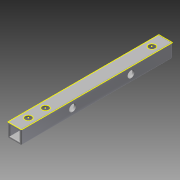
# Autodesk Inventor part: Vertical Rod
Saved by Autodesk Inventor 2013 (Build 170138000, 138)
## iProperties
Created: 2014-05-22
Part Number: Vertical Rod
Material: Steel
Document SubType Name: Modeling
Designer: ryclifton
Mass: 683.775 g
Surface Area: 479.026 cm^2
Volume: 87.105 cm^3
Density: 7.85 g/cm^3
Author: ryclifton
Autodesk Inventor part; units mm, degrees
ref_plane "YZ Plane" through (0, 0, 0) normal (1, 0, 0) x (0, 1, 0)
ref_plane "XZ Plane" through (0, 0, 0) normal (0, 1, 0) x (-1, 0, 0)
ref_plane "XY Plane" through (0, 0, 0) normal (0, 0, 1) x (1, 0, 0)
sketch "Sketch1" plane through (0, 0, 0) normal (0, 0, 1) x (1, 0, 0)
  line L0 (0, 0) -> (25.4, 0)
  line L1 (25.4, 0) -> (25.4, 25.4)
  line L2 (25.4, 25.4) -> (0, 25.4)
  line L3 (0, 25.4) -> (0, 0)
  dimension "d0" = 25.4
  dimension "d1" = 25.4
  constraints: 8 end point, 2 parallel, 1 horizontal, 1 perpendicular
  measures "d0" distance of L2.end L1.end
  measures "d1" distance of L1.end L0.end
extrude "Extrusion1" add sketch "Sketch1" along normal blind 279.4
sketch "Sketch2" plane through (0, 25.4, 0) normal (0, 1, 0) x (1, 0, 0)
  line L0 (0, 0) -> (0, -279.4) projected
  line L1 (25.4, 0) -> (25.4, -279.4) projected
  line L2 (0, 0) -> (0, -25.4)
  line L3 (0, -25.4) -> (12.7, -25.4)
  circle A0 centre (12.7, -25.4) radius 6.35
  line L4 (25.4, -279.4) -> (25.4, -254)
  line L5 (25.4, -254) -> (12.7, -254)
  circle A1 centre (12.7, -254) radius 6.35
  dimension "d4" = 25.4
  dimension "d5" = 12.7
  dimension "d6" = 25.4
  dimension "d7" = 12.7
  constraints: 8 end point, 2 centre point, 2 coincident, 2 perpendicular, 2 point on line
  measures "d4" distance of L0.start L2.end
  measures "d5" diameter of A0
  measures "d6" distance of L1.end L4.end
  measures "d7" diameter of A1
extrude "Extrusion2" cut sketch "Sketch2" against normal blind 279.4
sketch "Sketch3" plane through (0, 0, 0) normal (0, 0, -1) x (-1, 0, 0)
  line L0 (0, 0) -> (-25.4, 0) projected
  line L1 (-25.4, 25.4) -> (0, 25.4) projected
  line L2 (-25.4, 0) -> (-25.4, 25.4) projected
  line L3 (-25.4, 25.4) -> (-25.4, 21.59)
  line L4 (-25.4, 21.59) -> (-21.59, 21.59)
  line L5 (-25.4, 0) -> (-21.59, 0)
  line L6 (-21.59, 0) -> (-21.59, 3.81)
  line L7 (0, 0) -> (-3.81, 0)
  line L8 (-3.81, 0) -> (-3.81, 3.81)
  line L9 (0, 25.4) -> (-3.81, 25.4)
  line L10 (-3.81, 25.4) -> (-3.81, 21.59)
  line L11 (-3.81, 21.59) -> (-21.59, 21.59)
  line L12 (-21.59, 21.59) -> (-21.59, 3.81)
  line L13 (-21.59, 3.81) -> (-3.81, 3.81)
  line L14 (-3.81, 3.81) -> (-3.81, 21.59)
  dimension "d10" = 3.81
  dimension "d11" = 3.81
  dimension "d12" = 3.81
  dimension "d13" = 3.81
  dimension "d14" = 3.81
  dimension "d15" = 3.81
  dimension "d16" = 3.81
  dimension "d17" = 3.81
  constraints: 24 end point, 4 perpendicular, 4 point on line
  measures "d10" distance of L1.start L3.end
  measures "d11" distance of L3.end L4.end
  measures "d12" distance of L0.end L5.end
  measures "d13" distance of L5.end L6.end
  measures "d14" distance of L0.start L7.end
  measures "d15" distance of L7.end L8.end
  measures "d16" distance of L1.end L9.end
  measures "d17" distance of L9.end L10.end
extrude "Extrusion3" cut sketch "Sketch3" against normal blind 279.4 contours L13 L12 L11 L14
sketch "Sketch4" plane through (0, 0, 0) normal (0, -1, 0) x (1, 0, 0)
  circle A0 centre (12.7, 254) radius 6.35 projected
  line L0 (0, 0) -> (0, 279.4) projected
  line L1 (12.7, 247.65) -> (12.7, 222.25)
  circle A1 centre (12.7, 222.25) radius 6.35
  dimension "d20" = 25.4
  dimension "d21" = 12.7
  constraints: 2 end point, 1 centre point, 1 coincident, 1 parallel, 1 vertical alignment, 1 other
  measures "d20" distance of L1.start L1.end
  measures "d21" diameter of A1
extrude "Extrusion4" cut sketch "Sketch4" against normal blind 279.4 contours A1
sketch "Sketch5" plane through (0, 25.4, 0) normal (0, 1, 0) x (1, 0, 0)
  circle A0 centre (12.7, -222.25) radius 6.35 projected
  circle A1 centre (12.7, -25.4) radius 6.35 projected
  circle A2 centre (12.7, -254) radius 6.35 projected
  line L0 (25.4, 0) -> (0, 0) projected
  line L1 (0, 0) -> (0, -279.4) projected
  line L2 (25.4, -279.4) -> (0, -279.4) projected
  line L3 (25.4, 0) -> (25.4, -279.4) projected
sketch "Sketch6" plane through (25.4, 0, 0) normal (1, 0, 0) x (0, 0, -1)
  line L0 (0, 25.4) -> (-279.4, 25.4) projected
  line L1 (0, 0) -> (-279.4, 0) projected
  line L2 (-222.6507, 25.4) -> (-222.6507, 12.7)
  line L3 (-222.6507, 12.7) -> (-184.5507, 12.7)
  circle A0 centre (-184.5507, 12.7) radius 6.35
  line L4 (-178.2007, 12.7) -> (-76.6007, 12.7)
  circle A1 centre (-76.6007, 12.7) radius 6.35
  dimension "d25" = 12.7
  dimension "d24" = 38.1
  dimension "d26" = 101.6
  dimension "d27" = 12.7
  constraints: 6 end point, 2 coincident, 2 perpendicular, 1 centre point, 1 collinear, 1 horizontal alignment, 1 point on line, 2 other
  measures "d24" distance of L2.end L3.end
  measures "d26" distance of L4.start L4.end
  measures "d27" diameter of A1
extrude "Extrusion5" cut sketch "Sketch6" against normal blind 279.4
fillet "Fillet1" radius 1.5875 20 edges at (0, 0, 139.7) (0, 25.4, 139.7) (12.7, 25.4, 279.4) (12.7, 0, 279.4) (25.4, 12.7, 279.4) (0, 12.7, 279.4) (25.4, 25.4, 139.7) (25.4, 0, 139.7) (25.4, 12.7, 0) (12.7, 25.4, 0) (12.7, 21.59, 0) (3.81, 12.7, 0) (0, 12.7, 0) (12.7, 0, 0) (12.7, 3.81, 0) (21.59, 12.7, 0) (3.81, 12.7, 279.4) (12.7, 21.59, 279.4) (21.59, 12.7, 279.4) (12.7, 3.81, 279.4)
body "Solid1"
